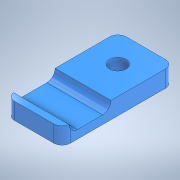
# Autodesk Inventor part: CableTieDown
Saved by Autodesk Inventor 2022 (Build 260153000, 153)
## iProperties
Created: 2022-02-22
Part Number: CableTieDown
Material: Generic
Document SubType Name: Modeling
Designer: Jorian Brusind
Density: 1 g/cm^3
Appearance: Cyan
Author: Jorian Brusind
Autodesk Inventor part; units mm, degrees
ref_plane "YZ Plane" through (0, 0, 0) normal (1, 0, 0) x (0, 1, 0)
ref_plane "XZ Plane" through (0, 0, 0) normal (0, 1, 0) x (-1, 0, 0)
ref_plane "XY Plane" through (0, 0, 0) normal (0, 0, 1) x (1, 0, 0)
sketch "Sketch1" plane through (0, 0, 0) normal (0, 1, 0) x (-1, 0, 0)
  line L0 (0, 0) -> (20, 0)
  line L1 (20, 0) -> (20, -40)
  line L2 (20, -40) -> (0, -40)
  line L3 (0, -40) -> (0, 0)
  circle A0 centre (10, -30) radius 3
  dimension "d0" = 20
  dimension "d1" = 40
  dimension "d2" = 6
  dimension "d3" = 10
  dimension "d4" = 10
  constraints: 8 end point, 2 parallel, 1 centre point, 1 horizontal, 1 perpendicular
  measures "d0" distance of L1.end L2.end
  measures "d1" distance of L0.end L1.end
  measures "d2" diameter of A0
  measures "d3" distance from line of L1 A0.centre
  measures "d4" distance from line of L2 A0.centre
extrude "Extrusion1" add sketch "Sketch1" along normal blind 6
sketch "Sketch2" plane through (0, 6, 0) normal (0, 1, 0) x (1, 0, 0)
  line L0 (-20, 0) -> (0, 0) projected
  line L1 (-10, 0) -> (-10, 10)
  line L2 (0, 17.5) -> (-20, 17.5)
  line L3 (-20, 17.5) -> (-20, 2.5)
  line L4 (-20, 2.5) -> (0, 2.5)
  line L5 (0, 2.5) -> (0, 17.5)
  line L6 (0, 17.5) -> (-20, 2.5) construction
  line L7 (-20, 17.5) -> (0, 2.5) construction
  dimension "d7" = 10
  dimension "d8" = 20
  dimension "d9" = 15
  constraints: 14 end point, 3 midpoint, 2 parallel, 1 horizontal, 1 perpendicular, 1 vertical
  measures "d7" distance of L1.start L1.end
  measures "d8" distance of L4.end L3.end
  measures "d9" distance of L3.end L2.end
extrude "Extrusion2" cut sketch "Sketch2" against normal blind 3
fillet "Fillet1" radius 3 2 edges at (-10, 3, -17.5) (-10, 3, -2.5)
fillet "Fillet2" radius 3 4 edges at (-20, 3, -40) (0, 3, -40) (-20, 3, 0) (0, 3, 0)
body "Solid1"
